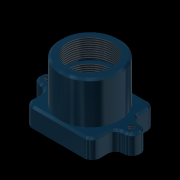
# Autodesk Inventor part: 3d_DAA - M12 Lens Mount
Saved by Autodesk Inventor 2018 (Build 220112000, 112)
## iProperties
Category: 0
Created: 2024-03-13
Part Number: 3d_DAA - M12 Lens Mount
Material: Aluminium 6061-T6
Document SubType Name: Modeling
Designer: cda1
Density: 2.7 g/cm^3
Appearance: Pantone 2965 U - Anodized
Mass: 4.08179 g
Surface Area: 21.2244 cm^2
Volume: 1.51178 cm^3
Manufacturer-1: {"Link": "", "Name": "SHENZHEN JINYIHE PROTOTYPE TECHNOLOGIES CO., LTD (JYH)", "PartNumber": "3d_DAA - M12 Lens Mount", "partner_id": false}
Manufacturer-2: {"Link": "", "Name": "QICHUANG MOLD CO., LTD", "PartNumber": "3d_DAA - M12 Lens Mount", "partner_id": false}
Manufacturer-3: {"Link": "", "Name": "SUNPE LIMITED", "PartNumber": "3d_DAA - M12 Lens Mount", "partner_id": false}
Manufacturer-4: {"Link": "", "Name": "", "PartNumber": "", "partner_id": false}
Manufacturer-5: {"Link": "", "Name": "", "PartNumber": "", "partner_id": false}
Provider-1: {"Link": "", "Name": "", "PartNumber": "", "partner_id": false}
Provider-2: {"Link": "", "Name": "", "PartNumber": "", "partner_id": false}
Provider-3: {"Link": "", "Name": "", "PartNumber": "", "partner_id": false}
Provider-4: {"Link": "", "Name": "", "PartNumber": "", "partner_id": false}
Provider-5: {"Link": "", "Name": "", "PartNumber": "", "partner_id": false}
odoo_id: 17986
odoo_internal_code: P010351
odoo_model: product.product
odoo_x2o_application_version: 12.0.4.10
odoo_d2o_version: 12.0.1.4.34
Author: cda1
Comments: DIN-2768-1-fine
Autodesk Inventor part; units mm, degrees
ref_plane "YZ Plane" through (0, 0, 0) normal (1, 0, 0) x (0, 1, 0)
ref_plane "XZ Plane" through (0, 0, 0) normal (0, 1, 0) x (-1, 0, 0)
ref_plane "XY Plane" through (0, 0, 0) normal (0, 0, 1) x (1, 0, 0)
sketch "Boceto1" plane through (0, 0, 0) normal (0, 0, 1) x (1, 0, 0)
  line L0 (-6.67, 7.35) -> (6.67, 7.35) construction
  line L1 (7.85, 6.17) -> (7.85, -6.17) construction
  line L2 (6.67, -7.35) -> (-6.67, -7.35) construction
  line L3 (-7.85, -6.17) -> (-7.85, 6.17) construction
  line L4 (-7.85, 7.35) -> (7.85, -7.35) construction
  line L5 (7.85, 7.35) -> (-7.85, -7.35) construction
  arc A0 (-7.85, -6.17) -> (-6.67, -7.35) centre (-6.67, -6.17) ccw construction
  arc A1 (-6.67, 7.35) -> (-7.85, 6.17) centre (-6.67, 6.17) ccw construction
  arc A2 (7.85, 6.17) -> (6.67, 7.35) centre (6.67, 6.17) ccw construction
  arc A3 (6.67, -7.35) -> (7.85, -6.17) centre (6.67, -6.17) ccw construction
  line L6 (-6.67, -8.35) -> (6.67, -8.35)
  arc A4 (6.67, -8.35) -> (8.85, -6.17) centre (6.67, -6.17) ccw
  line L7 (8.85, -6.17) -> (8.85, 6.17)
  arc A5 (8.85, 6.17) -> (6.67, 8.35) centre (6.67, 6.17) ccw
  line L8 (6.67, 8.35) -> (-6.67, 8.35)
  arc A6 (-6.67, 8.35) -> (-8.85, 6.17) centre (-6.67, 6.17) ccw
  line L9 (-8.85, 6.17) -> (-8.85, -6.17)
  arc A7 (-8.85, -6.17) -> (-6.67, -8.35) centre (-6.67, -6.17) ccw
  circle A8 centre (-11, 0) radius 0.8
  circle A9 centre (11, 0) radius 0.8
  arc A10 (11, -2.15) -> (11, 2.15) centre (11, 0) ccw
  arc A11 (-11, 2.15) -> (-11, -2.15) centre (-11, 0) ccw
  line L10 (-11, 2.15) -> (-8.85, 2.15)
  line L11 (-11, -2.15) -> (-8.85, -2.15)
  line L12 (11, 2.15) -> (8.85, 2.15)
  line L13 (11, -2.15) -> (8.85, -2.15)
  point P0 (0, 0)
  point P1 (0, 0)
  point P2 (0, 0)
  dimension "d0" = 15.7
  dimension "d1" = 14.7
  dimension "d2" = 1.18
  dimension "d3" = 2.18
  dimension "d9" = 1.6
  dimension "d10" = 1.6
  dimension "d11" = 22
  dimension "d12" = 11
  dimension "d13" = 4.3
  dimension "d14" = 4.3
  constraints: 28 end point, 20 point on circle, 16 point on line, 12 centre point, 10 tangent, 4 midpoint, 4 parallel, 4 perpendicular, 3 equal radius, 2 coincident, 2 horizontal alignment, 1 horizontal, 7 other
  measures "d0" distance of L4.end L5.end
  measures "d1" distance of L5.start L4.end
  measures "d2" radius of A0
  measures "d3" radius of A7
  measures "d9" diameter of A8
  measures "d10" diameter of A9
  measures "d11" distance of A8.centre A9.centre
  measures "d12" distance of point (0, 0) A9.centre
  measures "d13" diameter of A10
  measures "d14" diameter of A11
extrude "Extrusión1" add sketch "Boceto1" along normal blind 5 contours A7 L9 A6 L8 A5 L7 A4 L6 | L11 A11 L10 L9 | L7 L12 A10 L13 | A8 | A9
sketch "Boceto3" plane through (0, 0, 5) normal (0, 0, 1) x (1, 0, 0)
  circle A0 centre (0, 0) radius 7.8
  dimension "d15" = 15.6
  constraints: 1 centre point, 1 coincident
  measures "d15" diameter of A0
extrude "Extrusión3" add sketch "Boceto3" along normal blind 11
sketch "Boceto4" plane through (0, 0, 0) normal (0, 0, -1) x (-1, 0, 0)
  line L0 (-6.67, 7.35) -> (6.67, 7.35)
  line L1 (7.85, 6.17) -> (7.85, -6.17)
  line L2 (6.67, -7.35) -> (-6.67, -7.35)
  line L3 (-7.85, -6.17) -> (-7.85, 6.17)
  line L4 (-7.85, 7.35) -> (7.85, -7.35) construction
  line L5 (7.85, 7.35) -> (-7.85, -7.35) construction
  arc A0 (-6.67, 7.35) -> (-7.85, 6.17) centre (-6.67, 6.17) ccw
  arc A1 (-7.85, -6.17) -> (-6.67, -7.35) centre (-6.67, -6.17) ccw
  arc A2 (6.67, -7.35) -> (7.85, -6.17) centre (6.67, -6.17) ccw
  arc A3 (7.85, 6.17) -> (6.67, 7.35) centre (6.67, 6.17) ccw
  point P0 (0, 0)
  dimension "d18" = 15.7
  dimension "d19" = 14.7
  dimension "d20" = 1.18
  constraints: 12 end point, 8 point on circle, 8 point on line, 8 tangent, 4 centre point, 3 equal radius, 2 midpoint, 2 parallel, 1 horizontal, 1 perpendicular
  measures "d18" distance of L4.end L5.end
  measures "d19" distance of L5.start L4.end
  measures "d20" radius of A0
extrude "Extrusión4" cut sketch "Boceto4" against normal blind 4
sketch "Boceto5" plane through (0, 0, 16) normal (0, 0, 1) x (1, 0, 0)
  point P0 (0, 0)
hole "Agujero1" at (0, 0, 16) direction (0, 0, -1) diameter 11.459 end through all thread size "M12x0.5" class "6H" standard "ISO Metric profile"
sketch "Boceto6" plane through (0, 0, 5) normal (0, 0, 1) x (1, 0, 0)
  arc A0 (-11, 2.15) -> (-11, -2.15) centre (-11, 0) ccw construction
  arc A1 (11, -2.15) -> (11, 2.15) centre (11, 0) ccw construction
  point P0 (0, 0)
hole "Agujero2" at (-11, 0, 5) at (11, 0, 5) direction (0, 0, -1) diameter 1.567 end through all thread size "M2x0.4" class "6H" standard "ISO Metric profile"
chamfer "Chaflán1" distance 0.5 angle 45 1 edges at (-7.8, 0, 16)
fillet "Empalme1" radius 2 4 edges at (8.85, 2.15, 2.5) (8.85, -2.15, 2.5) (-8.85, 2.15, 2.5) (-8.85, -2.15, 2.5)
chamfer "Chaflán3" distance 0.5 angle 45 16 edges at (10.925, 2.15, 5) (13.15, 0, 5) (10.925, -2.15, 5) (8.85, -5.16, 5) (8.2115, -7.7115, 5) (0, -8.35, 5) (-8.2115, -7.7115, 5) (-8.85, -5.16, 5) (-10.925, -2.15, 5) (-13.15, 0, 5) (-10.925, 2.15, 5) (-8.85, 5.16, 5) (-8.2115, 7.7115, 5) (0, 8.35, 5) (8.2115, 7.7115, 5) (8.85, 5.16, 5)
sketch "Boceto9" plane through (0, 0, 0) normal (1, 0, 0) x (0, 1, 0)
  line L0 (-7.3, 16) -> (7.3, 16) construction
  line L1 (-7.8, 5) -> (7.8, 5) construction
  line L2 (-5.7295, 16) -> (5.7295, 16) construction
  line L3 (0, 16) -> (0, 5) construction
  arc A0 (6.25, 10) -> (6.25, 11) centre (6.25, 10.5) ccw
  line L4 (5.7295, 4) -> (5.7295, 16) construction
  line L5 (6.25, 11) -> (5.7295, 11)
  line L6 (6.25, 10) -> (5.7295, 10)
  line L7 (5.7295, 10) -> (5.7295, 11)
  line L8 (6.25, 10) -> (6.75, 10)
  line L9 (6.75, 10) -> (6.75, 11)
  line L10 (6.75, 11) -> (6.25, 11)
  point P0 (0, 0)
  dimension "d55" = 1
  dimension "d57" = 11.5
  dimension "d58" = 5.5
  constraints: 14 end point, 4 tangent, 3 midpoint, 2 perpendicular, 2 point on circle, 1 centre point, 1 collinear, 1 horizontal, 1 point on line
  measures "d55" diameter of A0
  measures "d58" distance from line of L0 A0.centre
revolve "Revolución1" cut sketch "Boceto9" angle 360 about axis through (0, 0, 16) along (0, 0, -1)
